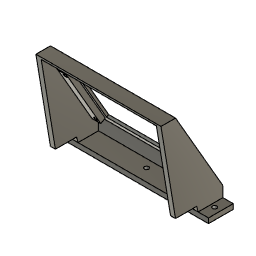
lcd_mount2 (Autodesk Fusion 360 design; units mm, degrees)
Autodesk Fusion 360 part; units mm, degrees
sketch "base drawings" plane through (0, 0, 0) normal (0, 0, 1) x (1, 0, 0)
  line L0 (60, 0) -> (-60, 0)
  line L1 (-60, 0) -> (-60, 20)
  line L2 (-60, 20) -> (60, 20)
  line L3 (60, 20) -> (60, 0)
  line L4 (66, 7) -> (-68, 7) construction
  line L5 (66, 13) -> (-68, 13) construction
  line L6 (-61, 3) -> (-61, 0)
  circle A0 centre (55, 10) radius 1.75
  circle A1 centre (-55, 10) radius 1.75
  circle A2 centre (0, 10) radius 1.75
  circle A3 centre (30, 15) radius 1.75
  circle A4 centre (-30, 15) radius 1.75
  line L7 (31.6743, 12.1) -> (33.3486, 15)
  line L8 (33.3486, 15) -> (31.6743, 17.9)
  line L9 (31.6743, 17.9) -> (28.3257, 17.9)
  line L10 (28.3257, 17.9) -> (26.6514, 15)
  line L11 (26.6514, 15) -> (28.3257, 12.1)
  line L12 (28.3257, 12.1) -> (31.6743, 12.1)
  line L13 (-28.3257, 12.1) -> (-26.6514, 15)
  line L14 (-26.6514, 15) -> (-28.3257, 17.9)
  line L15 (-28.3257, 17.9) -> (-31.6743, 17.9)
  line L16 (-31.6743, 17.9) -> (-33.3486, 15)
  line L17 (-33.3486, 15) -> (-31.6743, 12.1)
  line L18 (-31.6743, 12.1) -> (-28.3257, 12.1)
  line L19 (35, 20) -> (25, 20)
  line L20 (25, 20) -> (25, 10)
  line L21 (25, 10) -> (35, 10)
  line L22 (35, 10) -> (35, 20)
  line L23 (-25, 20) -> (-35, 20)
  line L24 (-35, 20) -> (-35, 10)
  line L25 (-35, 10) -> (-25, 10)
  line L26 (-25, 10) -> (-25, 20)
  line L27 (-35, 17.9) -> (-25, 17.9)
  line L28 (25, 17.9) -> (35, 17.9)
  point P0 (30, 15)
  point P1 (-30, 15)
  dimension "d1" = 120
  dimension "d2" = 20
  dimension "d52" = 3.5
  dimension "d53" = 3.5
  dimension "d54" = 3.5
  dimension "d55" = 3.5
  dimension "d56" = 3.5
  dimension "d57" = 2.9
  dimension "d58" = 2.9
  constraint perpendicular L3 L4
  constraint coincident L0 L6.end
  constraint perpendicular L0 L6
  constraint coincident P0 A3.centre
  constraint coincident P1 A4.centre
  constraint coincident L2 L19.start
  constraint coincident L2 L23.start
  constraint coincident L24 L27.start
  constraint coincident L26 L27.end
  constraint perpendicular L26 L27
  constraint coincident L20 L28.start
  constraint coincident L22 L28.end
  constraint perpendicular L22 L28
  measures "d1" distance of L0.start L0.end
  measures "d2" distance of L0.start L2.end
  measures "d52" diameter of A0
  measures "d53" diameter of A1
  measures "d54" diameter of A2
  measures "d55" diameter of A3
  measures "d56" diameter of A4
  measures "d57" distance of P0 L12
  measures "d58" distance of P1 L18
ref_plane "WorkPlane1" through (0, 20, 0) normal (0, 0.866025, 0.5) x (1, 0, 0)
sketch "screen1" plane through (12.125, 15, 8.6603) normal (0, 0.866025, 0.5) x (1, 0, 0)
  line L0 (20.5, 1) -> (20.5, -63)
  line L1 (35.5, -67) -> (32.5, -67)
  line L2 (35.5, 0) -> (35.5, -67)
  line L3 (32.5, -67) -> (32.5, 0)
  line L4 (18.5, 0) -> (18.5, -67)
  line L5 (-57.5, -57) -> (-57.5, 0)
  line L6 (-58.5, -3) -> (35.4087, -3)
  line L7 (-58.5, -53) -> (37.5, -53)
  line L8 (-57.5, 0) -> (32.5, 0)
  line L9 (32.5, 0) -> (35.5, 0)
  line L10 (-48, 1) -> (-48, -58.5616)
  line L11 (32.5, -67) -> (-57.5, -67)
  line L12 (32.5, 0) -> (32.5, -67)
  line L13 (29.5, -34) -> (28.5, -34)
  circle A0 centre (30.75, -52.5) radius 1.65
  line L14 (28.5, 1) -> (28.5, -57)
  line L15 (-52.75, -52.5) -> (-52.75, -3.5) construction
  line L16 (-50.5, 1) -> (-50.5, -58)
  circle A1 centre (30.75, -3.5) radius 1.65
  line L17 (30.75, -52.5) -> (-52.75, -52.5) construction
  line L18 (30.75, -3.5) -> (30.75, -52.5) construction
  line L19 (-52.75, -3.5) -> (30.75, -3.5) construction
  circle A2 centre (-52.75, -52.5) radius 1.65
  circle A3 centre (-52.75, -3.5) radius 1.65
  line L20 (29.5, -48) -> (29.5, -34)
  line L21 (28.5, -48) -> (29.5, -48)
  line L22 (-57.5, -55.5) -> (-57.5, -70)
  line L23 (-61.5, -70) -> (-61.5, 3)
  line L24 (32.5, 0) -> (32.5, 3)
  line L25 (32.5, -56) -> (32.5, -70)
  line L26 (39.5, 3) -> (39.5, -70)
  line L27 (-61.5, 3) -> (39.5, 3)
  line L28 (-57.5, 0) -> (-57.5, 3)
  line L29 (39.5, -70) -> (-61.5, -70)
  line L30 (28.5, -48) -> (32.5, -48)
  line L31 (32.5, -8.1885) -> (28.5, -8.1885)
  line L32 (32.5, -8.1885) -> (35.5, -8.1885)
  line L33 (32.5, -48) -> (35.5, -48)
  line L34 (-57.5, -57) -> (-50.5, -57)
  line L35 (28.5, -57) -> (35.5, -57)
  line L36 (35.5, -67) -> (35.5, -70)
  line L37 (-57.5, -57.0609) -> (32.5, -57)
  line L38 (24.3, -66.5) -> (19, -66.5)
  line L39 (19, -66.5) -> (19, -61.2)
  line L40 (19, -61.2) -> (24.3, -61.2)
  line L41 (24.3, -61.2) -> (24.3, -66.5)
  circle A4 centre (21.65, -63.85) radius 1.5
  line L42 (2, -61.2) -> (7.3, -61.2)
  line L43 (7.3, -61.2) -> (7.3, -66.5)
  line L44 (7.3, -66.5) -> (2, -66.5)
  circle A5 centre (4.65, -63.85) radius 1.5
  line L45 (2, -66.5) -> (2, -61.2)
  line L46 (-15, -61.2) -> (-9.7, -61.2)
  line L47 (-9.7, -61.2) -> (-9.7, -66.5)
  line L48 (-9.7, -66.5) -> (-15, -66.5)
  circle A6 centre (-12.35, -63.85) radius 1.5
  line L49 (-15, -66.5) -> (-15, -61.2)
  line L50 (-32, -61.2) -> (-26.7, -61.2)
  line L51 (-26.7, -61.2) -> (-26.7, -66.5)
  line L52 (-26.7, -66.5) -> (-32, -66.5)
  circle A7 centre (-29.35, -63.85) radius 1.5
  line L53 (-32, -66.5) -> (-32, -61.2)
  line L54 (-49, -61.2) -> (-43.7, -61.2)
  line L55 (-43.7, -61.2) -> (-43.7, -66.5)
  line L56 (-43.7, -66.5) -> (-49, -66.5)
  circle A8 centre (-46.35, -63.85) radius 1.5
  line L57 (-49, -66.5) -> (-49, -61.2)
  line L58 (19, -66.5) -> (24.3, -61.2) construction
  line L59 (24.3, -66.5) -> (19, -61.2) construction
  line L60 (27, -71) -> (27, -57)
  line L61 (-63, -69) -> (27, -69)
  line L62 (27, -59) -> (-57.5, -59)
  line L63 (-51.4429, -67) -> (-51.4429, -59)
  line L64 (-51.4429, -67) -> (-51.4429, -69)
  circle A9 centre (-55, -58) radius 0.9
  circle A10 centre (30, -58) radius 0.9
  line L65 (27, -59) -> (30, -60)
  line L66 (30, -60) -> (32.5, -59.8717)
  line L67 (27, -57) -> (26.9987, -55.051)
  line L68 (26.9987, -55.051) -> (32.5, -55.051)
  line L69 (-51.4429, -59) -> (-51.4429, -57)
  line L70 (-57.5, -55.5) -> (-51.4429, -55.5)
  line L71 (-51.4429, -55.5) -> (-51.4429, -57)
  line L72 (-51.4429, -55.5) -> (-50.5, -55.5)
  line L73 (32.5, -55.051) -> (35.5, -55.051)
  point P0 (21.65, -63.85)
  dimension "d16" = 90
  dimension "d24" = 83.5
  dimension "d25" = 49
  dimension "d26" = 3.3
  dimension "d27" = 3.3
  dimension "d28" = 3.3
  dimension "d29" = 3.3
  dimension "d140" = 3
  dimension "d143" = -17
  dimension "d144" = 0
  dimension "d163" = 5.3
  dimension "d164" = 5.3
  dimension "d165" = 1.8
  dimension "d166" = 1.8
  constraint horizontal L8
  constraint vertical L12
  constraint horizontal L11
  constraint vertical L5
  constraint coincident L4.start L8
  constraint coincident L4.end L11
  constraint perpendicular L4 L11
  constraint perpendicular L10 L11
  constraint perpendicular L6 L12
  constraint perpendicular L7 L10
  constraint perpendicular L0 L11
  constraint horizontal L9
  constraint vertical L2
  constraint horizontal L1
  constraint vertical L3
  constraint coincident L21.start L14
  constraint perpendicular L14 L21
  constraint coincident L13.end L14
  constraint perpendicular L13 L14
  constraint horizontal L19
  constraint vertical L18
  constraint horizontal L17
  constraint vertical L15
  constraint coincident L15.end L19.start
  constraint coincident A1.centre L18.start
  constraint coincident A0.centre L17.start
  constraint coincident L15.start L17.end
  constraint horizontal L27
  constraint vertical L26
  constraint horizontal L29
  constraint vertical L23
  constraint coincident L28.end L27
  constraint perpendicular L27 L28
  constraint coincident L24.end L27
  constraint perpendicular L24 L27
  constraint coincident L25.end L29
  constraint perpendicular L25 L29
  constraint coincident L22.end L29
  constraint perpendicular L22 L29
  constraint coincident L3 L30.end
  constraint perpendicular L3 L30
  constraint coincident L12 L31.start
  constraint coincident L14 L31.end
  constraint perpendicular L14 L31
  constraint coincident L2 L32.end
  constraint perpendicular L2 L32
  constraint coincident L2 L33.end
  constraint perpendicular L2 L33
  constraint coincident L16 L34.end
  constraint perpendicular L16 L34
  constraint coincident L2 L35.end
  constraint perpendicular L2 L35
  constraint coincident L29 L36.end
  constraint perpendicular L29 L36
  constraint coincident L22 L37.start
  constraint coincident L35 L37.end
  constraint coincident L12 L37.end
  constraint coincident L25 L37.end
  constraint horizontal L38
  constraint vertical L39
  constraint horizontal L40
  constraint vertical L41
  constraint midpoint L58 P0
  constraint vertical L60
  constraint coincident L60 L61.end
  constraint perpendicular L60 L61
  constraint coincident L60 L62.start
  constraint coincident L22 L62.end
  constraint perpendicular L22 L62
  constraint coincident L11 L63.start
  constraint coincident L62 L63.end
  constraint perpendicular L62 L63
  constraint coincident L61 L64.end
  constraint perpendicular L61 L64
  constraint coincident L25 L66.end
  constraint perpendicular L37 L67
  constraint coincident L12 L68.end
  constraint perpendicular L12 L68
  constraint coincident L34 L69.end
  constraint perpendicular L34 L69
  constraint perpendicular L69 L70
  constraint perpendicular L34 L71
  constraint coincident L16 L72.end
  constraint perpendicular L16 L72
  constraint coincident L2 L73.end
  constraint perpendicular L2 L73
  measures "d16" distance of L3.end L5.end
  measures "d24" distance of L15.end A1.centre
  measures "d25" distance of L15.end L15.start
  measures "d26" diameter of A3
  measures "d27" diameter of A1
  measures "d28" diameter of A0
  measures "d29" diameter of A2
  measures "d140" diameter of A4
  measures "d163" distance of L38.start L40.end
  measures "d164" distance of L39.end L40.end
  measures "d165" diameter of A9
  measures "d166" diameter of A10
extrude "Extrude1" add sketch "base drawings" along normal blind -8.5 and the other way blind 4.5 contours L0 L1 L2 L3 L20 L21 L22 L24 L25 L26 | L2 L9 L19 L20 L22 L28 | L2 L15 L23 L24 L26 L27 | L7 L8 L10 L11 L12 L20 L21 L22 L28 | L13 L14 L16 L17 L18 L24 L25 L26 L27 | L7 L8 L9 L10 L11 L12 L28 | L13 L14 L15 L16 L17 L18 L27 | A3 | A4 makes body 1
extrude "Extrude2" add sketch "screen1" along normal blind 2 separate body contours L0 L6 L8 L14 | L0 L4 L6 L8 | L8 L24 L27 L28 | L0 L6 L7 L14 | L0 L4 L6 L7 | L4 L6 L8 L10 | L3 L6 L8 L12 L14 A1 | L0 L7 L14 L37 L60 L67 L68 | L0 L4 L7 L37 | L3 L6 L12 L14 A1 L31 | L6 L8 L10 L16 | L2 L3 L9 L12 L32 | L2 L9 L24 L26 L27 L29 L36 | L0 L37 L60 L62 | L0 L4 L37 L62 | L4 L7 L10 L37 | L3 L7 L12 A0 L14 L21 L30 | L3 L7 L12 A0 L14 L68 | L6 L7 L10 L16 | L3 L12 L13 L14 L20 L30 L31 | L5 L6 L8 L16 A3 | L4 L11 L60 L62 | L4 L37 L62 L69 | L14 L35 L37 L60 L67 L68 | L3 L12 L25 L37 L60 L65 L66 | L7 L10 L16 L37 | L13 L14 L20 L21 L30 | L3 L12 L14 L25 L35 L68 | L5 L6 L7 L16 A2 A3 | L2 L3 L12 L32 L33 | L5 L22 L23 L27 L28 L61 | L3 L11 L12 L25 L60 L65 L66 | L4 L11 L62 L63 | L1 L2 L3 L12 L25 L35 | L2 L3 L12 L25 L35 L73 | L5 L7 L16 A2 L70 L72 | L2 L3 L7 L12 L73 | L2 L3 L7 L12 L33 | L11 L60 L61 L64 | L11 L25 L29 L60 | L11 L22 L62 L63 | L22 L37 L62 L69 | L16 L34 L37 L69 | L16 L34 L71 L72 | L22 L23 L29 L61 | L1 L25 L29 L36 | L22 L29 L60 L61 | L11 L22 L61 L64 | L22 L34 L37 L69 | L5 L22 L34 L70 L71 | L38 L39 L40 L41 | L42 L43 L44 L45 | L46 L47 L48 L49 | L50 L51 L52 L53 | L54 L55 L56 L57 | A9 | A10 makes body 2
extrude "Extrude4" add sketch "screen1" against normal blind 4.2 contours L3 L6 L8 L12 L14 A1 | L3 L6 L12 L14 A1 L31 | L2 L3 L9 L12 L32 | L3 L7 L12 A0 L14 L21 L30 | L3 L7 L12 A0 L14 L68 | L5 L6 L8 L16 A3 | L5 L6 L7 L16 A2 A3 | L5 L7 L16 A2 L70 L72 | L2 L3 L7 L12 L73 | L2 L3 L7 L12 L33 bodies 2
sketch "side" plane through (-49.375, 0, 0) normal (-1, 0, 0) x (0, -1, 0)
  line L0 (-16.5, 6.0622) -> (20, 69.282)
  line L1 (20, 69.282) -> (18.2679, 70.282)
  line L2 (18.2679, 70.282) -> (-18.2321, 7.0622)
  line L3 (-18.2321, 7.0622) -> (-16.5, 6.0622)
  line L4 (-18.2321, 7.0622) -> (18.2679, 70.282)
  line L5 (-20, -4.5) -> (-20, -8.5)
  line L6 (0, -4.5) -> (0, -8.5)
  line L7 (20, 69.282) -> (-16.5, 6.0622)
  line L8 (-15, 8.6603) -> (-11.3627, 6.5603)
  line L9 (16.3873, 54.6247) -> (-11.3627, 6.5603)
  line L10 (-18.2321, 7.0622) -> (-20, -4.5)
  line L11 (0, -4.5) -> (0, 41)
  line L12 (-20, -4.5) -> (0, -4.5)
  line L13 (-16.5, 6.0622) -> (-16.5, -4.5)
  line L14 (20, 69.282) -> (0, -4.5)
  line L15 (-16.0867, 10.778) -> (-22.4919, -0.3161)
  line L16 (-20, -4.5) -> (-20, 11)
  line L17 (-20, 0) -> (18.2679, 0)
  line L18 (18.2679, 0) -> (20, 69.282)
  line L19 (18.2679, 70.282) -> (30, 70.282)
  line L20 (30, 70.282) -> (18.2679, 0)
  line L21 (30, 68.5) -> (17.2391, 68.5)
  point P0 (-18.2321, 7.0622)
  constraint coincident P0 L2.end
  constraint coincident L5.start L10.end
  constraint coincident L6.start L11.start
  constraint vertical L11
  constraint coincident L0.start L3.end
  constraint coincident L12 L13.end
  constraint perpendicular L12 L13
  constraint coincident L0.end L1.start
  constraint coincident L2 L15.start
  constraint parallel L2 L15
  constraint vertical L16
  constraint coincident L16 L17.start
  constraint perpendicular L16 L17
  constraint coincident L1.end L2.start
  constraint horizontal L19
  constraint coincident L4 L21.end
  constraint horizontal L21
extrude "Extrude30" add sketch "side" against normal blind 4 contours L3 L10 L13 L17 | L0 L7 L8 L9 L11 L13 L17 | L0 L7 L8 L9 L11 | L10 L15 L16 L17 | L11 L12 L13 L17 | L10 L12 L13 L17 | L0 L7 L9 L11 L14 L21 | L10 L16 L17 | L11 L14 L17 | L9 L11 L14 L17 | L0 L7 L14 L21 | L14 L17 L18 L21 | L14 L18 L21 | L18 L20 L21 bodies 1 2
extrude "Extrude31" add sketch "side" along normal blind -97 and the other way blind 101 contours L3 L10 L13 L17 | L0 L7 L8 L9 L11 L13 L17 | L0 L7 L8 L9 L11 | L10 L15 L16 L17 | L11 L12 L13 L17 | L10 L12 L13 L17 | L0 L7 L9 L11 L14 L21 | L10 L16 L17 | L11 L14 L17 | L9 L11 L14 L17 | L0 L7 L14 L21 | L14 L17 L18 L21 | L14 L18 L21 | L18 L20 L21 bodies 1
extrude "Extrude32" add sketch "side" against normal blind 101 contours L3 L10 L13 L17 | L10 L15 L16 L17 | L10 L12 L13 L17 | L10 L16 L17 | L0 L1 L2 L4 L7 L21 | L1 L18 L19 L20 L21 bodies 1
extrude "Extrude34" add 1 faces at (-38.375, 4.5376, 23.9817) along direction (1, 0, 0) blind 90 and the other way blind -86 on bodies 1 bodies 1
extrude "Extrude35" add sketch "screen1" against normal blind 2.5 contours L2 L9 L24 L26 L27 L29 L36 | L4 L11 L60 L62 | L14 L35 L37 L60 L67 L68 | L3 L12 L25 L37 L60 L65 L66 | L3 L12 L14 L25 L35 L68 | L5 L22 L23 L27 L28 L61 | L4 L11 L62 L63 | L11 L60 L61 L64 | L11 L22 L62 L63 | L22 L37 L62 L69 | L22 L23 L29 L61 | L11 L22 L61 L64 | L22 L34 L37 L69 | L5 L22 L34 L70 L71 bodies 1
sketch "led_holder" plane through (0, 12.8349, 7.4103) normal (0, -0.866025, -0.5) x (1, 0, 0)
  line L0 (-45.375, 69) -> (-45.375, 55.5)
  line L1 (-45.375, 55.5) -> (-39.3179, 55.5)
  line L2 (-39.3179, 55.5) -> (-39.3179, 59)
  line L3 (-39.3179, 59) -> (39.125, 59)
  line L4 (39.125, 59) -> (39.125, 69)
  line L5 (39.125, 69) -> (-45.375, 69)
  line L6 (36.425, 61.2) -> (31.125, 61.2)
  line L7 (31.125, 61.2) -> (31.125, 66.5)
  line L8 (31.125, 66.5) -> (36.425, 66.5)
  line L9 (36.425, 66.5) -> (36.425, 61.2)
  circle A0 centre (-42.875, 58) radius 0.9
  line L10 (-19.875, 66.5) -> (-14.575, 66.5)
  line L11 (-14.575, 66.5) -> (-14.575, 61.2)
  line L12 (-14.575, 61.2) -> (-19.875, 61.2)
  line L13 (-19.875, 61.2) -> (-19.875, 66.5)
  line L14 (-36.875, 66.5) -> (-31.575, 66.5)
  line L15 (-31.575, 66.5) -> (-31.575, 61.2)
  line L16 (-31.575, 61.2) -> (-36.875, 61.2)
  line L17 (-36.875, 61.2) -> (-36.875, 66.5)
  line L18 (14.125, 66.5) -> (19.425, 66.5)
  line L19 (19.425, 66.5) -> (19.425, 61.2)
  line L20 (19.425, 61.2) -> (14.125, 61.2)
  line L21 (14.125, 61.2) -> (14.125, 66.5)
  line L22 (-2.875, 66.5) -> (2.425, 66.5)
  line L23 (2.425, 66.5) -> (2.425, 61.2)
  line L24 (2.425, 61.2) -> (-2.875, 61.2)
  line L25 (-2.875, 61.2) -> (-2.875, 66.5)
  line L26 (-39.3179, 59) -> (39.125, 59)
  line L27 (-39.3179, 55.5) -> (-39.3179, 59)
  circle A1 centre (-42.875, 58) radius 0.9
  circle A2 centre (-42.875, 58) radius 0.9
  circle A3 centre (42.125, 58) radius 0.9
  line L28 (39.125, 59) -> (39.125, 57)
  line L29 (39.125, 57) -> (39.1237, 55.051)
  line L30 (44.625, 55.051) -> (44.625, 59.8717)
  line L31 (39.125, 69) -> (-45.375, 69)
  line L32 (44.625, 59.8717) -> (44.625, 69)
  line L33 (44.625, 69) -> (39.125, 69)
  line L34 (-44.5394, 69) -> (-44.5394, 55.5)
  line L35 (-39.3179, 55.5) -> (-39.3179, 59)
  line L36 (39.1237, 55.051) -> (44.625, 55.051)
  line L37 (-44.5394, 55.5) -> (-39.3179, 55.5)
  circle A4 centre (-42.875, 58) radius 1.25
  circle A5 centre (42.125, 58) radius 1.25
  line L38 (39.125, 59) -> (39.125, 61)
  line L39 (44.625, 61) -> (39.125, 61)
  line L40 (-39.3179, 59) -> (-39.3179, 61.2)
  line L41 (-39.3179, 61.2) -> (-44.5394, 61.2)
  line L42 (-44.5394, 55.5) -> (-45.375, 55.5)
  line L43 (-45.375, 55.5) -> (-45.375, 69)
  line L44 (-44.5394, 61.2) -> (-45.375, 61.2)
  point P0 (39.125, 57)
  dimension "d167" = 2.5
  dimension "d168" = 2.5
  constraint coincident L30.end L32.start
  constraint perpendicular L31 L32
  constraint coincident L4.end L5.start
  constraint perpendicular L4 L33
  constraint coincident L5 L34.start
  constraint coincident L1 L34.end
  constraint perpendicular L1 L34
  constraint coincident L1.end L2.start
  constraint coincident L2.end L3.start
  constraint coincident L29.end L36.start
  constraint coincident L30.start L36.end
  constraint perpendicular L27 L37
  constraint concentric A0 A4
  constraint concentric A3 A5
  constraint coincident L3.end L4.start
  constraint coincident L4 L38.end
  constraint perpendicular L33 L38
  constraint coincident L32 L39.start
  constraint perpendicular L38 L39
  constraint perpendicular L26 L40
  constraint coincident L34 L41.end
  constraint perpendicular L34 L41
  constraint coincident L0.end L1.start
  constraint coincident L0.start L5.end
  constraint coincident L43 L44.end
  constraint perpendicular L43 L44
  measures "d167" diameter of A4
  measures "d168" diameter of A5
extrude "Extrude36" add sketch "led_holder" against normal blind 2 separate body contours L0 L5 L31 L34 L43 L44 | L0 L1 L34 L42 L43 L44 | L3 L4 L5 L26 L31 L34 L38 L40 L41 | L1 L2 L27 L34 L35 L37 L40 L41 | L4 L32 L33 L39 | L4 L28 L29 L30 L32 L36 L38 L39 | L6 L7 L8 L9 | L10 L11 L12 L13 | L14 L15 L16 L17 | L18 L19 L20 L21 | L22 L23 L24 L25 makes body 3
extrude "Extrude37" add sketch "led_holder" along normal blind 1.8 contours L0 L1 L34 L42 L43 L44 | L1 L2 L27 L34 L35 L37 L40 L41 | L4 L28 L29 L30 L32 L36 L38 L39 bodies 3
named bodies: "lcd_base", "lcd_shell", "led_holder"
